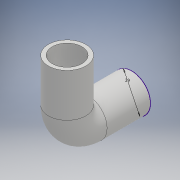
# Autodesk Inventor part: 90º Elbow
Saved by Autodesk Inventor 2017 (Build 210142000, 142)
## iProperties
Created: 2017-11-08
Part Number: 90º Elbow
Material: Generic
Document SubType Name: Modeling
Designer: DesignPC02
Density: 1 g/cm^3
Appearance: Default
Author: DesignPC02
Autodesk Inventor part; units mm, degrees
ref_plane "YZ Plane" through (0, 0, 0) normal (1, 0, 0) x (0, 1, 0)
ref_plane "Work Plane1" through (0, 0, 50) normal (0, 0, 1) x (1, 0, 0)
sketch "Sketch1" plane through (0, 0, 50) normal (0, 0, 1) x (1, 0, 0)
  circle A0 centre (0, 0) radius 14.5
  dimension "d1" = 29
  constraints: 1 centre point, 1 coincident
  measures "d1" diameter of A0
ref_plane "Work Plane2" through (0, 50, 0) normal (0, 1, 0) x (-1, 0, 0)
sketch "Sketch2" plane through (0, 50, 0) normal (0, 1, 0) x (-1, 0, 0)
  circle A0 centre (0, 0) radius 14.5
  dimension "d3" = 29
  constraints: 1 centre point, 1 coincident
  measures "d3" diameter of A0
sketch "Sketch3" plane through (0, 0, 0) normal (1, 0, 0) x (0, 1, 0)
  line L0 (50, -14.5) -> (50, 14.5) construction
  line L1 (14.5, 50) -> (-14.5, 50) construction
  line L2 (50, 0) -> (0, 0)
  line L3 (0, 50) -> (0, 0)
  line L4 (14.5, 50) -> (14.5, 16.5)
  line L5 (16.5, 14.5) -> (50, 14.5)
  arc A0 (14.5, 16.5) -> (16.5, 14.5) centre (16.5, 16.5) ccw
  dimension "d4" = 2
  constraints: 8 end point, 2 midpoint, 2 point on circle, 2 tangent, 1 centre point, 1 horizontal, 1 vertical, 1 other
  measures "d4" radius of A0
sweep "Sweep1" add profiles "Sketch1" path "Sketch3" path curves L4 A0 L5
shell "Shell1" thickness 3 removed faces 2 at (-0.6822, 50, 3.9778) at (-1.7139, -4.5192, 50)
body "Solid1"
